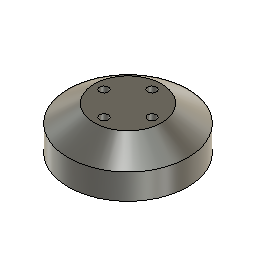
Adaptador JR3-HERRAMIENTA (Autodesk Fusion 360 design; units mm, degrees)
Autodesk Fusion 360 part; units mm, degrees
sketch "Boceto1" plane through (0, 0, 0) normal (0, 0, 1) x (1, 0, 0)
  circle A0 centre (0, 0) radius 31
  dimension "d1" = 62
  constraint coincident A0.centre origin
  measures "d1" diameter of A0
extrude "Extruir1" add sketch "Boceto1" along normal blind 12 makes body 1
sketch "Boceto2" plane through (0, 0, 12) normal (0, 0, 1) x (-1, 0, 0)
  circle A0 centre (0, 0) radius 31
  circle A1 centre (0, 0) radius 25
  circle A2 centre (0, -25) radius 3.1
  circle A3 centre (17.6777, -17.6777) radius 3.1
  circle A4 centre (25, 0) radius 3.1
  circle A5 centre (17.6777, 17.6777) radius 3.1
  circle A6 centre (0, 25) radius 3.1
  circle A7 centre (-17.6777, 17.6777) radius 3.1
  circle A8 centre (-25, 0) radius 3.1
  circle A9 centre (-17.6777, -17.6777) radius 3.1
  dimension "d4" = 50
  dimension "d5" = 6.2
  dimension "d7" = 360
  constraint concentric A0 A1
  constraint coincident A1 A2.centre
  measures "d4" diameter of A1
  measures "d5" diameter of A2
hole "Agujero1" at (-17.6777, 17.6777, 12) at (17.6777, 17.6777, 12) at (25, 0, 12) at (17.6777, -17.6777, 12) at (-17.6777, -17.6777, 12) at (-25, 0, 12) direction (0, 0, -1) diameter 6.5 depth 15 tip angle 180 counterbore diameter 11 counterbore depth 5 bodies 1
sketch "Boceto4" plane through (0, 0, 0) normal (0, 0, -1) x (1, 0, 0)
  circle A0 centre (-17.6777, 17.6777) radius 3.25
  circle A1 centre (17.6777, 17.6777) radius 3.25
  circle A2 centre (17.6777, -17.6777) radius 3.25
  circle A3 centre (-17.6777, -17.6777) radius 3.25
  circle A4 centre (25, 0) radius 3.25
  circle A5 centre (-25, 0) radius 3.25
  circle A6 centre (0, 0) radius 31
  circle A7 centre (0, 0) radius 25
  circle A8 centre (0, -25) radius 1
  circle A9 centre (9.5671, -23.097) radius 1
  circle A10 centre (17.6777, -17.6777) radius 1
  circle A11 centre (23.097, -9.5671) radius 1
  circle A12 centre (25, 0) radius 1
  circle A13 centre (23.097, 9.5671) radius 1
  circle A14 centre (17.6777, 17.6777) radius 1
  circle A15 centre (9.5671, 23.097) radius 1
  circle A16 centre (0, 25) radius 1
  circle A17 centre (-9.5671, 23.097) radius 1
  circle A18 centre (-17.6777, 17.6777) radius 1
  circle A19 centre (-23.097, 9.5671) radius 1
  circle A20 centre (-25, 0) radius 1
  circle A21 centre (-23.097, -9.5671) radius 1
  circle A22 centre (-17.6777, -17.6777) radius 1
  circle A23 centre (-9.5671, -23.097) radius 1
  dimension "d17" = 50
  dimension "d18" = 2
  dimension "d20" = 360
  constraint concentric A6 A7
  measures "d17" diameter of A7
  measures "d18" diameter of A8
hole "Agujero2" at (9.5671, 23.097, 0) at (-9.5671, 23.097, 0) at (9.5671, -23.097, 0) at (-9.5671, -23.097, 0) direction (0, 0, 1) diameter 4.5 depth 15 tip angle 180 counterbore diameter 5 counterbore depth 6 bodies 1
extrude "Extruir2" cut sketch "Boceto4" against normal blind 24 contours A7 A16 | A7 A16 bodies 1
delete_face "SuprimirCaras1" 1 faces at (-9.4549, 25.3442, 8) on bodies 1
delete_face "SuprimirCaras2" 1 faces at (9.6792, 25.3442, 8) on bodies 1
delete_face "SuprimirCaras3" 1 faces at (-9.4549, -20.8498, 8) on bodies 1
delete_face "SuprimirCaras4" 1 faces at (9.6792, -20.8498, 8) on bodies 1
delete_face "SuprimirCaras5" 1 faces at (0.995, -24.9004, 8) on bodies 1
delete_face "SuprimirCaras6" 1 faces at (-24.6764, -3.2339, 2.3333) on bodies 1
delete_face "SuprimirCaras7" 1 faces at (25.162, -3.246, 4.6667) on bodies 1
delete_face "SuprimirCaras8" 1 faces at (-24.4524, -5.4727, 8.6667) on bodies 1
delete_face "SuprimirCaras9" 1 faces at (25.5476, -5.4727, 8.6667) on bodies 1
extrude "Extruir3" cut 1 faces at (-4.6456, 4.5486, 12) along direction (0, 0, -1) blind 5 on bodies 1 bodies 1
extrude "Extruir4" add 1 faces at (-5.1557, -5.0984, 7) along direction (0, 0, 1) blind 6 on bodies 1 bodies 1
delete_face "SuprimirCaras10" 1 faces at (9.6917, -20.6001, 2) on bodies 1
delete_face "SuprimirCaras11" 1 faces at (9.6917, 25.5939, 2) on bodies 1
delete_face "SuprimirCaras12" 1 faces at (-9.4425, 25.5939, 2) on bodies 1
delete_face "SuprimirCaras13" 1 faces at (-9.4425, -20.6001, 2) on bodies 1
sketch "Boceto5" plane through (0, 0, 0) normal (1, 0, 0) x (0, 1, 0)
  line L0 (0, 14) -> (0, 19)
  line L1 (0, 19) -> (20, 19)
  line L2 (0, 14) -> (31, 14)
  line L3 (31, 14) -> (20, 19)
  dimension "d32" = 5
  dimension "d33" = 31
  dimension "d34" = 20
  dimension "d35" = 12.083
  constraint vertical L0
  constraint perpendicular L0 L1
  constraint perpendicular L0 L2
  measures "d32" distance of L0.start L0.end
  measures "d33" distance of L0.start L2.end
  measures "d34" distance of L0.end L1.end
  measures "d35" distance of L1.end L2.end
revolve "Revolución1" add sketch "Boceto5" angle 360 about axis through (0, 0, 14) along (0, 0, 1) separate body makes body 2
move_body "Desplazar1" bodies 2 to x (1, 0, 0) y (0, 1, 0) z (0, 0, 1) at (0, 0, -1)
move_body "Desplazar2" bodies 1 2 to x (1, 0, 0) y (0, 1, 0) z (0, 0, 1) at (0, -95, 0)
sketch "Boceto6" plane through (0, 0, 0) normal (0, 0, 1) x (1, 0, 0)
  circle A0 centre (0, 0) radius 20
  circle A1 centre (0, 12.5) radius 2
  circle A2 centre (-12.5, 0) radius 2
  circle A3 centre (12.5, 0) radius 2
  circle A4 centre (0, -12.5) radius 2
  dimension "d38" = 4
  constraint coincident A0.centre origin
  measures "d38" diameter of A1
extrude "Extruir5" add sketch "Boceto6" along normal blind 6 separate body makes body 3
move_body "Desplazar3" bodies 3 to x (1, 0, 0) y (0, 1, 0) z (0, 0, 1) at (0, -95, 18)
hole "Agujero3" at (0, -82.5, 18) direction (0, 0, -1) diameter 5.6 depth 20 tip angle 180 bodies 1 2
hole "Agujero4" at (0, -107.5, 18) direction (0, 0, -1) diameter 5.6 depth 20 tip angle 180 bodies 1 2
hole "Agujero5" at (12.5, -95, 18) direction (0, 0, -1) diameter 5.6 depth 20 tip angle 180 bodies 1 2
hole "Agujero6" at (-12.5, -95, 18) direction (0, 0, -1) diameter 5.6 depth 20 tip angle 180 bodies 1 2
move_body "Desplazar4" bodies 3 to x (1, 0, 0) y (0, 1, 0) z (0, 0, 1) at (62, 0, 0)
hole "Agujero7" at (17.6777, -77.3223, 0) direction (0, 0, 1) diameter 8 depth 13 tip angle 180 bodies 1
hole "Agujero8" at (17.6777, -112.6777, 0) direction (0, 0, 1) diameter 8 depth 13 tip angle 180 bodies 1
hole "Agujero9" at (-17.6777, -112.6777, 0) direction (0, 0, 1) diameter 8 depth 13 tip angle 180 bodies 1
hole "Agujero10" at (-17.6777, -77.3223, 0) direction (0, 0, 1) diameter 8 depth 13 tip angle 180 bodies 1
sketch "Boceto7" plane through (0, 0, 0) normal (0, 0, 1) x (1, 0, 0)
  circle A0 centre (0, 0) radius 15.5
  dimension "d65" = 31
  constraint coincident A0.centre origin
  measures "d65" diameter of A0
extrude "Extruir6" add sketch "Boceto7" against normal blind 10 separate body makes body 4
move_body "Desplazar5" bodies 4 to x (1, 0, 0) y (0, 1, 0) z (0, 0, 1) at (0, 70, 0)
move_body "Desplazar6" bodies 2 1 to x (1, 0, 0) y (0, 1, 0) z (0, 0, 1) at (0, 90, 0)
move_body "Desplazar7" bodies 1 2 to x (1, 0, 0) y (0, 1, 0) z (0, 0, 1) at (0, 5, 0)
move_body "Desplazar8" bodies 4 to x (1, 0, 0) y (0, 1, 0) z (0, 0, 1) at (0, -70, 0)
extrude "Extruir7" cut 1 faces at (3.6156, 2.7614, -10) along direction (0, 0, 1) blind 16.5 on bodies 4 bodies 1 4
sketch "Boceto8" plane through (0, 0, 0) normal (0, 0, 1) x (1, 0, 0)
  circle A0 centre (-26.5, 0) radius 2.5
  dimension "d70" = 5
  measures "d70" diameter of A0
sketch "Boceto9" plane through (0, 0, 0) normal (0, 0, 1) x (1, 0, 0)
extrude "Extruir8" add sketch "Boceto8" against normal blind 5 separate body makes body 5
move_body "Desplazar9" bodies 5 to x (1, 0, 0) y (0, 1, 0) z (0, 0, 1) at (2, 0, 0)
extrude "Extruir9" cut 1 faces at (-24.7589, 0.6598, -5) along direction (0, 0, 1) blind 2 on bodies 5 bodies 5
sketch "Boceto10" plane through (0, 0, 0) normal (0, 1, 0) x (1, 0, 0)
extrude "Extruir10" cut 1 faces at (-24.7589, 0.6598, -3) along direction (0, 0, 1) blind 9 on bodies 5 bodies 1 5
hole "Agujero11" at (12.5, 0, 6.5) direction (0, 0, 1) diameter 7 depth 2 tip angle 180 bodies 1
hole "Agujero12" at (12.5, 0, 0) direction (0, 0, 1) diameter 7 depth 6.5 tip angle 180 bodies 1
hole "Agujero13" at (0, 12.5, 0) direction (0, 0, 1) diameter 7 depth 2 tip angle 180 bodies 1
hole "Agujero14" at (0, 12.5, 0) direction (0, 0, 1) diameter 7 depth 6.5 tip angle 180 bodies 1
hole "Agujero15" at (0, 12.5, 6.5) direction (0, 0, 1) diameter 7 depth 2 tip angle 180 bodies 1
hole "Agujero16" at (-12.5, 0, 6.5) direction (0, 0, 1) diameter 7 depth 2 tip angle 180 bodies 1
hole "Agujero17" at (0, -12.5, 6.5) direction (0, 0, 1) diameter 7 depth 2 tip angle 180 bodies 1
hole "Agujero18" at (-12.5, 0, 0) direction (0, 0, 1) diameter 7 depth 6.5 tip angle 180 bodies 1
hole "Agujero19" at (0, -12.5, 0) direction (0, 0, 1) diameter 7 depth 6.5 tip angle 180 bodies 1
delete_face "SuprimirCaras14" 1 faces at (0.1396, 9.7035, 11.5) on bodies 1
delete_face "SuprimirCaras15" 1 faces at (12.6396, -2.7965, 11.5) on bodies 1
delete_face "SuprimirCaras16" 1 faces at (-12.3604, -2.7965, 11.5) on bodies 1
delete_face "SuprimirCaras17" 1 faces at (0.1396, -15.2965, 11.5) on bodies 1
hole "Agujero20" at (12.5, 0, 8.5) direction (0, 0, 1) diameter 4 depth 6.5 tip angle 180 bodies 1
hole "Agujero21" at (0, 12.5, 8.5) direction (0, 0, 1) diameter 4 depth 6.5 tip angle 180 bodies 1
hole "Agujero22" at (0, -12.5, 8.5) direction (0, 0, 1) diameter 4 depth 6.5 tip angle 180 bodies 1
hole "Agujero23" at (-12.5, 0, 8.5) direction (0, 0, 1) diameter 4 depth 6.5 tip angle 180 bodies 1
extrude "Extruir11" add sketch "Boceto8" against normal blind 12 separate body makes body 6
sketch "Boceto11" plane through (0, 0, 0) normal (0, 1, 0) x (1, 0, 0)
delete_face "SuprimirCaras18" 1 faces at (-22.0124, 0.2489, 2) on bodies 1
move_face "MoveFace1" to x (1, 0, 0) y (0, 1, 0) z (0, 0, 1) at (1.5, 0, 0) 1 faces at (-24.0031, -0.1246, -8) on bodies 6
extrude "Extruir12" cut 1 faces at (-25.2589, 0.6598, -12) along direction (0, 0, 1) blind 18 on bodies 6 bodies 1 6
delete_face "SuprimirCaras19" 1 faces at (0.0997, 14.4975, 10) on bodies 1
delete_face "SuprimirCaras20" 1 faces at (12.5997, 1.9975, 10) on bodies 1
delete_face "SuprimirCaras21" 1 faces at (-12.4003, 1.9975, 10) on bodies 1
delete_face "SuprimirCaras22" 1 faces at (0.0997, -10.5025, 10) on bodies 1
hole "Agujero24" at (0, 12.5, 8.5) direction (0, 0, 1) diameter 4.5 depth 6.5 tip angle 180 bodies 1
hole "Agujero25" at (-12.5, 0, 8.5) direction (0, 0, 1) diameter 4.5 depth 6.5 tip angle 180 bodies 1
hole "Agujero26" at (12.5, 0, 8.5) direction (0, 0, 1) diameter 4.5 depth 6.5 tip angle 180 bodies 1
hole "Agujero27" at (0, -12.5, 8.5) direction (0, 0, 1) diameter 4.5 depth 6.5 tip angle 180 bodies 1
hole "Agujero28" at (-25, 0, 0) direction (0, 0, 1) diameter 6 depth 6 tip angle 180 bodies 1
extrude "Extruir13" add 1 faces at (8.3554, -21.426, 0) along direction (0, 0, -1) blind 0.2 on bodies 1 bodies 1 4 5 6
hole "Agujero29" at (0, 12.5, 6.5) direction (0, 0, 1) diameter 8 depth 3 tip angle 180 bodies 1
hole "Agujero30" at (0, 12.5, -0.2) direction (0, 0, 1) diameter 8 depth 8.7 tip angle 180 bodies 1
hole "Agujero31" at (-12.5, 0, -0.2) direction (0, 0, 1) diameter 8 depth 8.7 tip angle 180 bodies 1
hole "Agujero32" at (0, -12.5, -0.2) direction (0, 0, 1) diameter 8 depth 8.7 tip angle 180 bodies 1
hole "Agujero33" at (12.5, 0, -0.2) direction (0, 0, 1) diameter 8 depth 8.7 tip angle 180 bodies 1
hole "Agujero34" at (12.5, 0, 6.5) direction (0, 0, 1) diameter 8 depth 3 tip angle 180 bodies 1
hole "Agujero35" at (0, -12.5, 6.5) direction (0, 0, 1) diameter 8 depth 3 tip angle 180 bodies 1
hole "Agujero36" at (-12.5, 0, 6.5) direction (0, 0, 1) diameter 8 depth 3 tip angle 180 bodies 1
hole "Agujero37" at (-12.5, 0, 6.5) direction (0, 0, 1) diameter 8 depth 4 tip angle 180 bodies 1
hole "Agujero38" at (0, 12.5, 6.5) direction (0, 0, 1) diameter 8 depth 4 tip angle 180 bodies 1
hole "Agujero39" at (0, -12.5, 6.5) direction (0, 0, 1) diameter 8 depth 4 tip angle 180 bodies 1
hole "Agujero40" at (12.5, 0, 6.5) direction (0, 0, 1) diameter 8 depth 4 tip angle 180 bodies 1
hole "Agujero41" at (-25, 0, -0.2) direction (0, 0, 1) diameter 7 depth 6.2 tip angle 180 bodies 1
hole "Agujero42" at (0, -12.5, 6.5) direction (0, 0, 1) diameter 8 depth 6.7 tip angle 180 bodies 1 2
delete_face "SuprimirCaras23" 1 faces at (12.6396, -2.7965, 16.3333) on bodies 2
delete_face "SuprimirCaras24" 1 faces at (0.1396, -15.2965, 16.4) on bodies 2
hole "Agujero43" at (0, -12.5, 13.2) direction (0, 0, 1) diameter 4.5 depth 8 tip angle 180 bodies 2
sketch "Boceto12" plane through (0, 0, 0) normal (1, 0, 0) x (0, 1, 0)
  line L0 (0, 40) -> (0, 49)
  line L1 (0, 49) -> (17.5, 49)
  line L2 (17.5, 49) -> (31, 40)
  line L3 (31, 40) -> (0, 40)
  constraint vertical L0
  constraint perpendicular L0 L1
  constraint perpendicular L0 L3
revolve "Revolución2" add sketch "Boceto12" angle 360 about axis through (0, 0, 40) along (0, 0, 1) separate body makes body 7
move_body "Desplazar10" bodies 7 to x (1, 0, 0) y (0, 1, 0) z (0, 0, 1) at (0, 0, -18)
move_body "Desplazar11" bodies 7 to x (1, 0, 0) y (0, 1, 0) z (0, 0, 1) at (0, 0, -9)
hole "Agujero44" at (17.6777, -17.6777, -0.2) direction (0, 0, 1) diameter 8.5 depth 13.2 tip angle 180 bodies 1
hole "Agujero45" at (17.6777, 17.6777, -0.2) direction (0, 0, 1) diameter 8.5 depth 13.2 tip angle 180 bodies 1
hole "Agujero46" at (-17.6777, -17.6777, -0.2) direction (0, 0, 1) diameter 8.5 depth 13.2 tip angle 180 bodies 1
hole "Agujero47" at (-17.6777, 17.6777, -0.2) direction (0, 0, 1) diameter 8.5 depth 13.2 tip angle 180 bodies 1
move_body "Desplazar12" bodies 7 to x (1, 0, 0) y (0, 1, 0) z (0, 0, 1) at (0, 0, 20)
move_body "Desplazar13" bodies 7 to x (1, 0, 0) y (0, 1, 0) z (0, 0, 1) at (0, 0, -20)
hole "Agujero48" at (0, -12.5, 13) direction (0, 0, 1) diameter 4.5 depth 13.2 tip angle 180 bodies 7
hole "Agujero49" at (12.5, 0, 13) direction (0, 0, 1) diameter 4.5 depth 13.2 tip angle 180 bodies 7
hole "Agujero50" at (0, 12.5, 13) direction (0, 0, 1) diameter 4.5 depth 13.2 tip angle 180 bodies 7
hole "Agujero51" at (-12.5, 0, 13) direction (0, 0, 1) diameter 4.5 depth 13.2 tip angle 180 bodies 7
hole "Agujero52" at (12.5, 0, 6.5) direction (0, 0, 1) diameter 8 depth 6.7 tip angle 180 bodies 1 7
hole "Agujero53" at (0, 12.5, 6.5) direction (0, 0, 1) diameter 8 depth 6.7 tip angle 180 bodies 1 7
hole "Agujero54" at (-12.5, 0, 6.5) direction (0, 0, 1) diameter 8 depth 6.7 tip angle 180 bodies 1 7
hole "Agujero55" at (0, -12.5, 6.5) direction (0, 0, 1) diameter 8 depth 6.7 tip angle 180 bodies 7
hidden bodies 2 3
